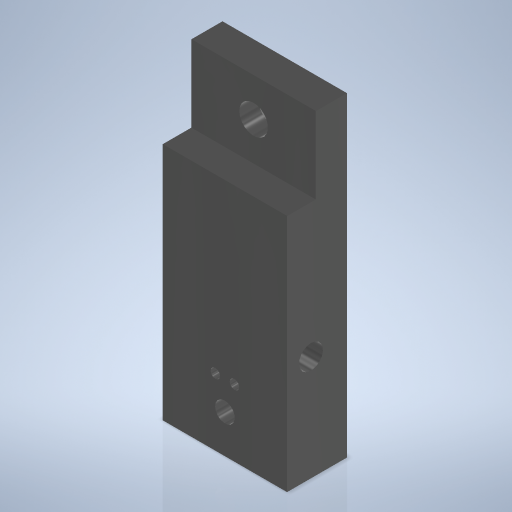
# Autodesk Inventor part: support
Saved by Autodesk Inventor 2024 (Build 280153000, 153)
## iProperties
Created: 2024-06-06
Part Number: support
Material: Aluminium 6061
Document SubType Name: Modeling
Designer: ffogue
Density: 2.7 g/cm^3
Appearance: Dunkelgrau
Author: ffogue
Autodesk Inventor part; units mm, degrees
note: some values were not read from the file. Chosen so that the rebuilt part matches the saved one: direction of "Bohrung1"; direction of "Bohrung2"; direction of "Bohrung3".
ref_plane "YZ Plane" through (0, 0, 0) normal (1, 0, 0) x (0, 1, 0)
ref_plane "XZ Plane" through (0, 0, 0) normal (0, 1, 0) x (-1, 0, 0)
ref_plane "XY Plane" through (0, 0, 0) normal (0, 0, 1) x (1, 0, 0)
sketch "Skizze1" plane through (0, 0, 0) normal (0, 1, 0) x (-1, 0, 0)
  line L0 (13, 0) -> (-13, 0)
  line L1 (-13, 0) -> (-13, 66)
  line L2 (-13, 66) -> (13, 66)
  line L3 (13, 66) -> (13, 0)
  point P0 (0, 0)
  point P1 (0, 0)
  dimension "d0" = 66
  dimension "d1" = 26
  constraints: 8 end point, 2 parallel, 1 coincident, 1 horizontal, 1 midpoint, 1 perpendicular
  measures "d0" distance between parallel lines of L0 L2
  measures "d1" distance between parallel lines of L1 L3
extrude "Extrusion1" add sketch "Skizze1" along normal blind 13
sketch "Skizze2" plane through (-13, 0, 0) normal (-1, 0, 0) x (0, 0, 1)
  line L0 (66, 0) -> (66, 13) projected
  line L1 (66, 6) -> (50, 6)
  line L2 (0, 13) -> (66, 13) projected
  line L3 (50, 6) -> (50, 0)
  line L4 (50, 0) -> (66, 0)
  line L5 (66, 6) -> (66, 0)
  point P0 (0, 0)
  dimension "d4" = 7
  dimension "d5" = 16
  constraints: 8 end point, 1 collinear, 1 horizontal, 1 perpendicular, 1 point on line, 1 vertical
  measures "d4" distance between parallel lines of L1 L2
  measures "d5" distance between parallel lines of L3 L0
extrude "Extrusion2" cut sketch "Skizze2" against normal up to surface (26 mm away)
sketch "Skizze3" plane through (0, 13, 0) normal (0, 1, 0) x (1, 0, 0)
  line L0 (-13, -66) -> (13, -66) projected
  line L1 (13, 0) -> (-13, 0) projected
  point P0 (0, 0)
  point P1 (0, -58)
  point P2 (0, 0)
  dimension "d8" = 8
  constraints: 1 midpoint, 1 vertical alignment
  measures "d8" distance from line of L0 point (0, -58)
hole "Bohrung1" at (0, 13, 58) direction (0, -1, 0) diameter 6 depth 7 countersink diameter 12 countersink angle 90
sketch "Skizze4" plane through (0, 13, 0) normal (0, 1, 0) x (1, 0, 0)
  line L0 (13, 0) -> (-13, 0) projected
  point P0 (0, 0)
  point P1 (0, -8)
  point P2 (0, 0)
  point P3 (0, 0)
  dimension "d23" = 8
  constraints: 2 midpoint, 1 vertical alignment
  measures "d23" distance of point (0, 0) point (0, -8)
hole "Bohrung2" at (0, 13, 8) direction (0, -1, 0) diameter 4.134 depth 13 thread size "M5x0.8" class "6H" standard "ISO Metric profile"
sketch "Skizze5" plane through (0, 13, 0) normal (0, 1, 0) x (1, 0, 0)
  line L0 (13, 0) -> (-13, 0) projected
  point P0 (0, 0)
  point P1 (2, -14)
  point P2 (-2, -14)
  point P3 (0, 0)
  point P4 (0, 0)
  dimension "d31" = 2
  dimension "d32" = 2
  dimension "d33" = 14
  dimension "d34" = 14
  constraints: 2 midpoint
  measures "d31" horizontal distance of point (0, 0) point (2, -14)
  measures "d32" horizontal distance of point (0, 0) point (-2, -14)
  measures "d33" distance from line of L0 point (2, -14)
  measures "d34" distance from line of L0 point (-2, -14)
hole "Bohrung3" at (2, 13, 14) at (-2, 13, 14) direction (0, -1, 0) diameter 2 depth 13
sketch "Skizze6" plane through (-13, 0, 0) normal (-1, 0, 0) x (0, 0, 1)
  line L0 (0, 0) -> (50, 0) projected
  point P0 (22, 10.5)
  point P1 (22, 5)
  dimension "d42" = 22
  dimension "d43" = 5
  dimension "d44" = 5.5
  constraints: 1 vertical alignment
  measures "d42" horizontal distance of L0.start point (22, 5)
  measures "d43" distance from line of L0 point (22, 5)
  measures "d44" distance of point (22, 5) point (22, 10.5)
hole "Bohrung4" at (-13, 5, 22) direction (1, 0, 0) diameter 4.134 depth 13 counterbore diameter 5 counterbore depth 6 thread size "M5x0.8" class "6H" standard "ISO Metric profile"
hole "Bohrung5" at (-13, 10.5, 22) direction (1, 0, 0) diameter 2 depth 13
mirror "Spiegeln1" about plane through (0, 0, 0) normal (1, 0, 0) of "Bohrung4"
chamfer "Fasen1" distance 0.5 angle 45 4 edges at (-13, 13, 33) (0, 13, 66) (13, 13, 33) (0, 13, 0)
sketch "Skizze7" plane through (13, 0, 0) normal (0, 0, -1) x (-1, 0, 0)
  line L0 (0, 0) -> (0, 12.5) projected
  line L1 (0, 0) -> (26, 0) projected
  point P0 (13, 0)
  point P1 (5, 6.5)
  point P2 (21, 6.5)
  point P3 (0, 6.25)
  point P4 (0, 6.25)
  dimension "d62" = 5
  dimension "d63" = 16
  dimension "d64" = 6.5
  constraints: 2 midpoint, 1 horizontal alignment
  measures "d62" horizontal distance of point (0, 6.25) point (5, 6.5)
  measures "d63" distance of point (21, 6.5) point (5, 6.5)
  measures "d64" distance from line of L1 point (5, 6.5)
hole "Bohrung6" at (8, 6.5, 0) at (-8, 6.5, 0) direction (0, 0, 1) diameter 4.917 depth 15 thread size "M6x1" class "6H" standard "ISO Metric profile"
